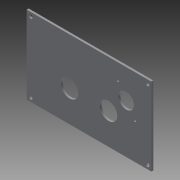
# Autodesk Inventor part: Gearbox plate
Saved by Autodesk Inventor 2015 (Build 190159000, 159)
## iProperties
Created: 2015-01-28
Part Number: Gearbox plate
Material: Generic
Document SubType Name: Modeling
Designer: whitaus15
Density: 1 g/cm^3
Appearance: Default
Author: whitaus15
Autodesk Inventor part; units mm, degrees
ref_plane "YZ Plane" through (0, 0, 0) normal (1, 0, 0) x (0, 1, 0)
ref_plane "XZ Plane" through (0, 0, 0) normal (0, 1, 0) x (-1, 0, 0)
sketch "Sketch1" plane through (0, 0, 0) normal (0, 0, 1) x (1, 0, 0)
  line L0 (0, 0) -> (-203.2, 0)
  line L1 (-203.2, 0) -> (-203.2, 127)
  line L2 (-203.2, 127) -> (0, 127)
  line L3 (0, 127) -> (0, 0)
  dimension "d0" = 127
  dimension "d1" = 203.2
  constraints: 8 end point, 2 parallel, 1 horizontal, 1 perpendicular
  measures "d0" distance of L2.end L0.start
  measures "d1" distance of L0.start L0.end
extrude "Extrusion1" add sketch "Sketch1" along normal blind 3.175
sketch "Sketch2" plane through (0, 0, 3.175) normal (0, 0, 1) x (1, 0, 0)
  circle A0 centre (-69.85, 50.8) radius 14.2875
  line L0 (0, 0) -> (0, 127) projected
  line L1 (-203.2, 0) -> (0, 0) projected
  circle A1 centre (-133.35, 50.8) radius 14.2875
  line L2 (-101.6, 0) -> (-101.6, 50.8)
  line L3 (-101.6, 50.8) -> (-69.85, 50.8)
  line L4 (-69.85, 50.8) -> (-133.35, 50.8)
  dimension "d4" = 28.575
  dimension "d8" = 28.575
  dimension "d9" = 50.8
  dimension "d28" = 63.5
  dimension "d29" = 31.75
  constraints: 6 end point, 2 centre point, 1 collinear, 1 horizontal, 1 midpoint, 1 vertical
  measures "d4" diameter of A0
  measures "d8" diameter of A1
  measures "d9" distance from line of L1 L4.end
  measures "d28" distance of L3.end L4.end
  measures "d29" distance of L2.end L3.end
extrude "Extrusion2" cut sketch "Sketch2" against normal blind 3.175
sketch "Sketch3" plane through (0, 0, 3.175) normal (0, 0, 1) x (1, 0, 0)
  circle A0 centre (-6.35, 6.35) radius 3.175
  line L0 (0, 0) -> (0, 127) projected
  line L1 (-203.2, 0) -> (0, 0) projected
  circle A1 centre (-6.35, 120.65) radius 3.175
  line L2 (0, 127) -> (-203.2, 127) projected
  circle A2 centre (-196.85, 120.65) radius 3.175
  circle A3 centre (-196.85, 6.35) radius 3.175
  line L3 (-203.2, 127) -> (-203.2, 0) projected
  dimension "d12" = 6.35
  dimension "d13" = 6.35
  dimension "d14" = 6.35
  dimension "d15" = 6.35
  dimension "d16" = 6.35
  dimension "d17" = 6.35
  dimension "d18" = 6.35
  dimension "d19" = 6.35
  dimension "d20" = 6.35
  dimension "d30" = 6.35
  dimension "d31" = 6.35
  dimension "d32" = 6.35
  constraints: 4 centre point
  measures "d12" diameter of A0
  measures "d13" distance from line of L0 A0.centre
  measures "d14" distance from line of L1 A0.centre
  measures "d15" diameter of A1
  measures "d16" distance from line of L0 A1.centre
  measures "d17" distance from line of L2 A1.centre
  measures "d18" diameter of A2
  measures "d19" distance from line of A2.centre L2
  measures "d20" diameter of A3
  measures "d30" distance from line of A2.centre L3
  measures "d31" distance from line of L3 A3.centre
  measures "d32" distance from line of L1 A3.centre
hole "Hole1" at (-196.85, 120.65, 3.175) at (-196.85, 6.35, 3.175) at (-6.35, 6.35, 3.175) at (-6.35, 120.65, 3.175) direction (0, 0, -1) diameter 6.35 end through all
ref_plane "Work Plane1" through (-101.6, 0, 0) normal (1, 0, 0) x (0, 0, -1)
sketch "Sketch4" plane through (0, 0, 3.175) normal (0, 0, 1) x (1, 0, 0)
  circle A0 centre (-69.85, 50.8) radius 14.2875 projected
  line L0 (-69.85, 50.8) -> (-41.0234, 79.6266)
  line L1 (-69.85, 50.8) -> (-23.1148, 50.8)
  circle A1 centre (-41.0234, 79.6266) radius 12.7
  point P0 (0, 0)
  dimension "d33" = 40.767
  dimension "d34" = 315
  dimension "d35" = 25.4
  constraints: 4 end point, 1 centre point, 1 coincident, 1 horizontal
  measures "d33" distance of L0.start L0.end
  measures "d35" diameter of A1
extrude "Extrusion3" cut sketch "Sketch4" against normal through all contours A1
sketch "Sketch5" plane through (0, 0, 3.175) normal (0, 0, 1) x (1, 0, 0)
  circle A0 centre (-41.0234, 79.6266) radius 12.7 projected
  line L0 (-41.0234, 79.6266) -> (-27.001, 58.448)
  line L1 (-41.0234, 79.6266) -> (-19.8448, 93.649)
  line L2 (-41.0234, 79.6266) -> (-55.0458, 100.8052)
  circle A1 centre (-55.0458, 100.8052) radius 1.9844
  circle A2 centre (-19.8448, 93.649) radius 1.9844
  circle A3 centre (-27.001, 58.448) radius 1.9844
  point P0 (0, 0)
  dimension "d38" = 25.4
  dimension "d39" = 25.4
  dimension "d40" = 25.4
  dimension "d41" = 3.9688
  dimension "d42" = 3.9688
  dimension "d43" = 3.9688
  constraints: 6 end point, 3 centre point, 3 coincident, 1 perpendicular, 1 point on line
  measures "d38" distance of L0.start L0.end
  measures "d39" distance of L0.start L1.end
  measures "d40" distance of L0.start L2.end
  measures "d41" diameter of A1
  measures "d42" diameter of A2
  measures "d43" diameter of A3
extrude "Extrusion4" cut sketch "Sketch5" against normal blind 25.4 contours A3 | A1
equation "\"d29\" = 0.5 * d28"
body "Solid1"
